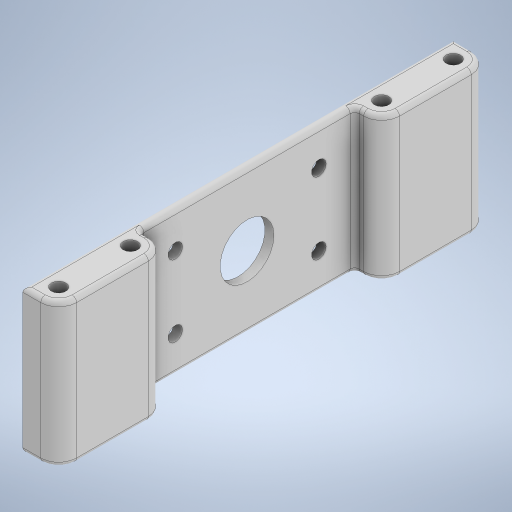
# Autodesk Inventor part: Connector plate
Saved by Autodesk Inventor 2023 (Build 270158000, 158)
## iProperties
Created: 2023-02-07
Part Number: Connector plate
Material: Generic
Document SubType Name: Modeling
Designer: Gabriel - T3 CAD
Density: 1 g/cm^3
Appearance: Default
Author: Gabriel - T3 CAD
Autodesk Inventor part; units mm, degrees
ref_plane "YZ Plane" through (0, 0, 0) normal (1, 0, 0) x (0, 1, 0)
ref_plane "XZ Plane" through (0, 0, 0) normal (0, 1, 0) x (-1, 0, 0)
ref_plane "XY Plane" through (0, 0, 0) normal (0, 0, 1) x (1, 0, 0)
sketch "Sketch1" plane through (0, 0, 0) normal (0, 1, 0) x (-1, 0, 0)
  line L0 (0, 0) -> (-3.175, 0)
  line L1 (-3.175, 0) -> (-3.175, 101.6)
  line L2 (-3.175, 101.6) -> (0, 101.6)
  line L3 (0, 101.6) -> (0, 0)
  line L4 (0, 0) -> (-3.175, 0)
  line L5 (-3.175, 0) -> (-3.175, -25.4)
  line L6 (-3.175, -25.4) -> (0, -25.4)
  line L7 (0, -25.4) -> (0, 0)
  line L8 (0, 101.6) -> (-3.175, 101.6)
  line L9 (-3.175, 101.6) -> (-3.175, 127)
  line L10 (-3.175, 127) -> (0, 127)
  line L11 (0, 127) -> (0, 101.6)
  circle A0 centre (-6.35, 120.65) radius 2.5797
  circle A1 centre (-6.35, 95.25) radius 2.5797
  line L12 (0, 127) -> (-12.7, 127)
  line L13 (-12.7, 127) -> (-12.7, 88.9)
  line L14 (-12.7, 88.9) -> (0, 88.9)
  line L15 (0, 88.9) -> (0, 127)
  line L16 (25.4, 50.8) -> (-25.4, 50.8)
  line L17 (25.4, 50.8) -> (76.2, 50.8) construction
  line L18 (-3.175, 101.6) -> (-3.175, 0)
  line L19 (-3.175, 0) -> (0, 0)
  line L20 (0, 0) -> (0, 101.6)
  line L21 (0, 0) -> (-3.175, 0)
  line L22 (-3.175, 0) -> (-3.175, -25.4)
  line L23 (-3.175, -25.4) -> (0, -25.4)
  line L24 (0, -25.4) -> (0, 0)
  circle A2 centre (-6.35, -19.05) radius 2.5797
  circle A3 centre (-6.35, 6.35) radius 2.5797
  line L25 (0, -25.4) -> (-12.7, -25.4)
  line L26 (-12.7, -25.4) -> (-12.7, 12.7)
  line L27 (-12.7, 12.7) -> (0, 12.7)
  line L28 (0, 12.7) -> (0, -25.4)
  circle A4 centre (-6.35, 6.35) radius 6.35
  circle A5 centre (-6.35, -19.05) radius 6.35
  circle A6 centre (-6.35, 95.25) radius 6.35
  circle A7 centre (-6.35, 120.65) radius 6.35
  point P0 (-3.175, 88.9)
  point P1 (-3.175, 12.7)
  point P2 (-12.7, -19.05)
  point P3 (0, -19.05)
  point P4 (0, 120.65)
  point P5 (-3.175, 115.1507)
  point P6 (-3.175, 100.7493)
  point P7 (-6.35, 88.9)
  point P8 (-6.35, 12.7)
  point P9 (-12.7, 6.35)
  point P10 (-6.35, 127)
  point P11 (-12.7, 120.65)
  point P12 (-12.7, 95.25)
  point P13 (-6.35, -25.4)
  dimension "d25" = 3.175
  dimension "d26" = 101.6
  dimension "d27" = 3.175
  dimension "d28" = 25.4
  dimension "d29" = 3.175
  dimension "d30" = 25.4
  dimension "d31" = 0
  dimension "d32" = 25.4
  dimension "d33" = 6.35
  dimension "d34" = 5.1594
  dimension "d35" = 5.1594
  dimension "d36" = 12.7
  dimension "d37" = 38.1
  dimension "d38" = 6.35
  dimension "d39" = 50.8
  dimension "d40" = 180
  dimension "d41" = 50.8
  dimension "d42" = 25.4
  constraints: 58 end point, 10 symmetric about line, 8 centre point, 8 parallel, 5 horizontal, 4 coincident, 4 perpendicular, 2 tangent, 1 collinear, 2 other
  measures "d25" distance of L1.end L2.end
  measures "d26" distance of L0.end L1.end
  measures "d27" distance of L6.end L5.end
  measures "d28" distance of L5.end L4.end
  measures "d29" distance of L9.end L10.end
  measures "d30" distance of L8.end L9.end
  measures "d31" horizontal distance of A0.centre A1.centre
  measures "d32" distance of A0.centre A1.centre
  measures "d33" distance from line of A0.centre L10
  measures "d34" diameter of A1
  measures "d35" diameter of A0
  measures "d36" distance of L14.end L13.end
  measures "d37" distance of L13.end L12.end
  measures "d38" distance from line of L15 A0.centre
  measures "d39" distance of L16.start L16.end
  measures "d40" angle of L16 L17
  measures "d41" distance from line of L0.start L16
  measures "d42" distance from line of L3 L16.start
extrude "Extrusion1" add sketch "Sketch1" along normal blind 50.8 contours L7 A5 L5 L0 | L0 L1 A4 L3 | L5 A5 L26 A4 L1 | A4 L1 L27 L3 | A4 L1 | A5 L5 | L7 L6 L5 A5 | A4 L1 | L5 A5 | L27 L1 L16 L3 | A4 L27 L1 | L5 L25 A5 | L16 L1 L14 L3 | L14 L1 A6 L3 | A6 L1 L2 L3 | A6 L1 | L14 A6 L1 | L2 L9 A7 L11 | A6 L13 A7 L9 L1 | L1 A6 | A7 L9 L10 L11 | A7 L9 | A7 L9 | A7 L12 L9
sketch "Sketch3" plane through (3.175, 0, 88.9) normal (1, 0, 0) x (0, 0, -1)
  circle A0 centre (12.7, 12.7) radius 2.5797
  line L0 (0, 0) -> (76.2, 0)
  line L1 (0, 0) -> (0, 50.8)
  circle A1 centre (63.5, 12.7) radius 2.5797
  circle A2 centre (12.7, 38.1) radius 2.5797
  circle A3 centre (63.5, 38.1) radius 2.5797
  circle A4 centre (38.1, 25.4) radius 9.525
  point P0 (88.9, 0)
  dimension "d43" = 12.7
  dimension "d44" = 12.7
  dimension "d45" = 5.1594
  dimension "d48" = 50.8
  dimension "d51" = 25.4
  dimension "d56" = 19.05
  dimension "d57" = 25.4
  dimension "d58" = 38.1
  constraints: 5 centre point, 4 end point, 1 horizontal, 1 vertical, 6 other
  measures "d43" distance from line of L0 A0.centre
  measures "d44" distance from line of L1 A0.centre
  measures "d45" diameter of A0
  measures "d48" distance of A0.centre A1.centre
  measures "d51" distance of A0.centre A2.centre
  measures "d56" diameter of A4
  measures "d57" distance from line of L0 A4.centre
  measures "d58" distance from line of L1 A4.centre
extrude "Extrusion3" cut sketch "Sketch3" against normal blind 50.8
fillet "Fillet3" radius 1.5875 26 edges at (0, 50.8, 50.8) (0, 0, 50.8) (10.8401, 50.8, 125.1401) (12.7, 50.8, 107.95) (10.8401, 50.8, 90.7599) (4.7625, 50.8, 88.9) (3.175, 50.8, 127) (10.8401, 0, 125.1401) (12.7, 0, 107.95) (10.8401, 0, 90.7599) (4.7625, 0, 88.9) (3.175, 0, 127) (3.175, 25.4, 88.9) (3.175, 50.8, 50.8) (3.175, 50.8, -25.4) (12.7, 50.8, -6.35) (10.8401, 50.8, 10.8401) (4.7625, 50.8, 12.7) (10.8401, 50.8, -23.5401) (3.175, 0, -25.4) (12.7, 0, -6.35) (10.8401, 0, 10.8401) (4.7625, 0, 12.7) (10.8401, 0, -23.5401) (3.175, 0, 50.8) (3.175, 25.4, 12.7)
equation "\"d35\" = d34"
body "Solid1"
